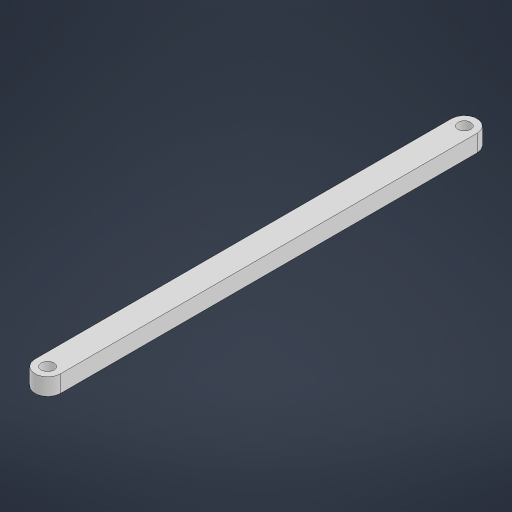
# Autodesk Inventor part: MainBar
Saved by Autodesk Inventor 2024.2 (Build 282272000, 272)
## iProperties
Created: 2023-12-28
Part Number: MainBar
Material: 一般
Document SubType Name: Modeling
Designer: Hanaoka
Density: 1 g/cm^3
Appearance: 既定
Author: Hanaoka
Autodesk Inventor part; units mm, degrees
ref_plane "YZ Plane" through (0, 0, 0) normal (1, 0, 0) x (0, 1, 0)
ref_plane "XZ Plane" through (0, 0, 0) normal (0, 1, 0) x (-1, 0, 0)
ref_plane "XY Plane" through (0, 0, 0) normal (0, 0, 1) x (1, 0, 0)
sketch "スケッチ1" plane through (0, 0, 0) normal (0, 1, 0) x (-1, 0, 0)
  line L0 (0, 52) -> (0, 52)
  line L1 (3, 49) -> (3, -49)
  line L2 (0, -52) -> (0, -52)
  line L3 (-3, -49) -> (-3, 49)
  line L4 (-3, 52) -> (3, -52) construction
  line L5 (3, 52) -> (-3, -52) construction
  arc A0 (0, -52) -> (3, -49) centre (0, -49) ccw
  arc A1 (-3, -49) -> (0, -52) centre (0, -49) ccw
  arc A2 (0, 52) -> (-3, 49) centre (0, 49) ccw
  arc A3 (3, 49) -> (0, 52) centre (0, 49) ccw
  circle A4 centre (0, 49) radius 1.5
  circle A5 centre (0, 49) radius 3 construction
  line L6 (3, 0) -> (-3, 0) construction
  circle A6 centre (0, -49) radius 1.5
  circle A7 centre (0, -49) radius 3 construction
  point P0 (0, 0)
  dimension "d0" = 3
  dimension "d2" = 6
  dimension "d3" = 3
  dimension "d4" = 6
  dimension "d10" = 98
  constraints: 14 end point, 10 tangent, 8 centre point, 8 point on circle, 8 point on line, 4 midpoint, 3 equal radius, 2 coincident, 2 parallel, 2 symmetric about line, 1 horizontal, 1 perpendicular, 2 other
  measures "d0" radius of A0
  measures "d2" distance between parallel lines of L3 L1
  measures "d3" diameter of A4
  measures "d4" diameter of A5
  measures "d10" distance of A6.centre A4.centre
extrude "押し出し1" add sketch "スケッチ1" along normal blind 4
